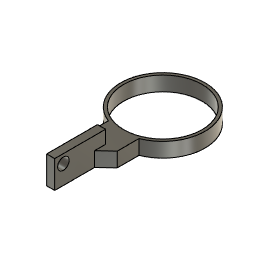
Holder v4 (Autodesk Fusion 360 design; units mm, degrees)
Autodesk Fusion 360 part; units mm, degrees
note: some values were not read from the file. Chosen so that the rebuilt part matches the saved one: which face or edge a step refers to.
sketch "Sketch1" plane through (0, 0, 0) normal (1, 0, 0) x (0, 1, 0)
  circle A0 centre (0, 0) radius 29
  circle A1 centre (0, 0) radius 27
  line L0 (-42, 10.583) -> (-27, 10.583)
  line L1 (-27, 10.583) -> (-27, -10.583)
  line L2 (-27, -10.583) -> (-42, -10.583)
  line L3 (-42, -10.583) -> (-42, 10.583)
  line L4 (-42, 3.0423) -> (-77, 3.0423)
  line L5 (-77, 3.0423) -> (-77, -2.5177)
  line L6 (-77, -2.5177) -> (-42, -2.5177)
  line L7 (-42, -2.5177) -> (-42, 3.0423)
  line L8 (-42, 3.0423) -> (-77, -2.5177) construction
  line L9 (-77, 3.0423) -> (-42, -2.5177) construction
  point P0 (-59.5, 0.2623)
  dimension "d1" = 58
  dimension "d3" = 54
  dimension "d4" = 15
  dimension "d5" = 5.56
  dimension "d6" = 35
  constraint coincident A0.centre A1.centre
  constraint concentric A0 A1
  constraint horizontal L0
  constraint vertical L1
  constraint horizontal L2
  constraint vertical L3
  constraint tangent A1 L1
  constraint coincident A0 L1.end
  constraint coincident A0 L0.end
  constraint horizontal L4
  constraint perpendicular L4 L5
  constraint parallel L4 L6
  constraint parallel L5 L7
  constraint coincident L3 L4.start
  constraint coincident L8 P0
  constraint coincident L9 P0
  measures "d1" diameter of A0
  measures "d3" diameter of A1
  measures "d4" distance of L0.start L0.end
  measures "d5" distance of L4.end L5.end
  measures "d6" distance of L4.start L4.end
extrude "Extrude1" add sketch "Sketch1" along normal blind 5 contours A0 L1 | A0 L1 | A0 L0 L2 L3 L7
extrude "Extrude2" add sketch "Sketch1" along normal blind 9 contours L3 L4 L5 L6 L7
hole "Hole2" at (4.5, -69, 3.0423) direction (0, 0, -1) diameter 6 depth 50 tip angle 118
sketch "Sketch4" plane through (0, 0, 0) normal (-1, 0, 0) x (0, -1, 0)
  circle A0 centre (0, 0) radius 27
  arc A1 (27, 10.583) -> (27, -10.583) centre (0, 0) ccw
  line L0 (27, -10.583) -> (42, -10.583)
  line L1 (42, -10.583) -> (42, -2.5177)
  line L2 (42, -2.5177) -> (77, -2.5177)
  line L3 (77, -2.5177) -> (77, 3.0423)
  line L4 (77, 3.0423) -> (42, 3.0423)
  line L5 (42, 3.0423) -> (42, 10.583)
  line L6 (42, 10.583) -> (27, 10.583)
  line L7 (42, 10.583) -> (49.5509, 3.0423)
  line L8 (49.5509, -2.5177) -> (42, -10.583)
  constraint coincident L5.end L6.start
  constraint coincident L4 L7.end
  constraint coincident L2 L8.start
  constraint coincident L0.end L1.start
extrude "Extrude4" add sketch "Sketch4" against normal blind 5 contours L4 L5 L7 | L1 L2 L8
move_body "Move2" bodies 1 to x (0, 0, 1) y (0, 1, 0) z (-1, 0, 0) at (7.5423, 0, -1.4577)
extrude "Extrude5" add 1 faces at (7.5423, -37, -1.4577) along direction (0, 0, -1) blind 5
move_face "MoveFace1" to x (1, 0, 0) y (0, 0.5, 0.866025) z (0, -0.866025, 0.5) at (0, -31.7774, 58.2782) 1 faces at (6.3533, -71.9963, 3.1918)
delete_face "DeleteFace1" 1 faces at (6.3533, -69.2852, 3.0203)
extrude "Extrude6" add 1 faces at (6.3533, -65.3333, 7.5423) along direction (0, 0, 1) blind 5
sketch "Sketch5" plane through (10.06, 0, 0) normal (1, 0, 0) x (0, 1, 0)
  line L0 (-49.5509, 3.5423) -> (-42, 3.5423)
  line L1 (-42, 3.5423) -> (-42, 12.5423)
  line L2 (-42, 12.5423) -> (-77, 12.5423)
  line L3 (-77, 12.5423) -> (-77, -6.4577)
  line L4 (-77, -6.4577) -> (-49.5509, -6.4577)
  line L5 (-49.5509, -6.4577) -> (-49.5509, 3.5423)
  line L6 (-71, 12.5423) -> (-71, -6.4577)
  line L7 (-77, 6.5423) -> (-42, 6.5423)
  circle A0 centre (-71, 6.5423) radius 4
  dimension "d29" = 6
  dimension "d30" = 6
  dimension "d31" = 8
  constraint coincident L2 L6.start
  constraint coincident L4 L6.end
  constraint perpendicular L4 L6
  constraint coincident L3 L7.start
  constraint perpendicular L6 L7
  constraint coincident L6 A0.centre
  constraint coincident L7 A0.centre
  measures "d29" distance of L2 L7
  measures "d30" distance of L3 L6
  measures "d31" diameter of A0
hole "Hole3" at (10.06, -71, 6.5423) direction (-1, 0, 0) diameter 8 depth 8 tip angle 118
hole "Hole1" [suppressed]
move_body "Move1" [suppressed]
sketch "Sketch3" plane through (0, 0, -4.8892) normal (0, 0, -1) x (1, 0, 0)
  circle A0 centre (5.1108, 0) radius 27
  arc A1 (-5.4722, 27) -> (15.6938, 27) centre (5.1108, 0) ccw
  line L0 (15.6938, 27) -> (15.6938, 42)
  line L1 (15.6938, 42) -> (7.6285, 42)
  line L2 (7.6285, 42) -> (7.6285, 61)
  line L3 (7.6285, 61) -> (2.0685, 61)
  line L4 (2.0685, 61) -> (2.0685, 42)
  line L5 (2.0685, 42) -> (-5.4722, 42)
  line L6 (-5.4722, 42) -> (-5.4722, 27)
  line L7 (-5.4722, 42) -> (2.0685, 48.4019)
  line L8 (15.6938, 42) -> (7.6285, 48.4019)
  constraint coincident L5.end L6.start
  constraint coincident L4 L7.end
  constraint coincident L0.end L1.start
  constraint coincident L2 L8.end
extrude "Extrude3" [suppressed]
